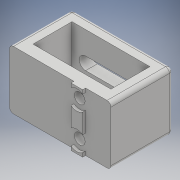
# Autodesk Inventor part: Estrutura - Suporte Mesa
Saved by Autodesk Inventor 2017 (Build 210142000, 142)
## iProperties
Created: 2020-08-23
Part Number: Estrutura - Suporte Mesa
Material: Generic
Document SubType Name: Modeling
Designer: ale
Density: 1 g/cm^3
Appearance: Default
Author: ale
Autodesk Inventor part; units mm, degrees
note: some values were not read from the file. Chosen so that the rebuilt part matches the saved one: direction of "Hole1".
ref_plane "YZ Plane" through (0, 0, 0) normal (1, 0, 0) x (0, 1, 0)
ref_plane "XZ Plane" through (0, 0, 0) normal (0, 1, 0) x (-1, 0, 0)
ref_plane "XY Plane" through (0, 0, 0) normal (0, 0, 1) x (1, 0, 0)
sketch "Sketch1" plane through (0, 0, 0) normal (0, 0, 1) x (1, 0, 0)
  line L0 (-12.2491, 0) -> (12.2491, 0)
  line L1 (0, 10.917) -> (0, -10.917)
  line L2 (-30, -10) -> (-30, -16)
  line L3 (-30, -16) -> (16, -16)
  line L4 (-30, -10) -> (10, -10)
  line L5 (10, -10) -> (10, 10)
  line L6 (10, 10) -> (-30, 10)
  line L7 (-30, 10) -> (-30, 16)
  line L8 (-30, 16) -> (16, 16)
  line L9 (16, 16) -> (16, -16)
  point P0 (0, 0)
  point P1 (0, 0)
  dimension "d0" = 10
  dimension "d1" = 10
  dimension "d2" = 10
  dimension "d3" = 30
  dimension "d4" = 6
  dimension "d5" = 6
  dimension "d6" = 40
  dimension "d7" = 6
  constraints: 20 end point, 6 perpendicular, 2 horizontal, 2 midpoint, 2 vertical, 1 coincident
  measures "d0" distance between parallel lines of L6 L0
  measures "d1" distance between parallel lines of L4 L0
  measures "d2" distance between parallel lines of L5 L1
  measures "d3" distance between parallel lines of L2 L1
  measures "d4" distance between parallel lines of L3 L4
  measures "d5" distance between parallel lines of L9 L5
  measures "d6" distance between parallel lines of L7 L5
  measures "d7" distance between parallel lines of L6 L8
extrude "Extrusion1" add sketch "Sketch1" along normal blind 30 contours L5 L6 L7 L8 L9 L3 L2 L4
sketch "Sketch2" plane through (-30, -16, 0) normal (0, -1, 0) x (1, 0, 0)
  line L0 (40, 30) -> (0, 30) projected
  line L1 (27, 30) -> (27, 0)
  line L2 (0, 0) -> (0, 30) projected
  line L3 (33, 30) -> (33, 0)
  line L4 (40, 0) -> (0, 0) projected
  line L5 (27, 30) -> (33, 30)
  line L6 (33, 0) -> (27, 0)
  line L7 (46, 0) -> (46, 30) projected
  line L8 (40, 0) -> (40, 30) projected
  point P0 (30, 0)
  dimension "d37" = 13
  dimension "d38" = 7
  constraints: 8 end point, 3 point on line, 2 collinear, 1 perpendicular, 1 vertical
  measures "d37" distance between parallel lines of L8 L1
  measures "d38" distance between parallel lines of L8 L3
extrude "Extrusion2" add sketch "Sketch2" along normal blind 1.5 contours L3 L4 L1 L0
sketch "Sketch3" plane through (-30, -17.5, 0) normal (0, -1, 0) x (1, 0, 0)
  line L0 (27, 0) -> (33, 0) projected
  line L1 (27, 30) -> (27, 0) projected
  line L2 (27, 15) -> (13, 15)
  line L3 (33, 0) -> (33, 30) projected
  point P0 (30, 0)
  point P1 (30, 6)
  point P2 (30, 24)
  dimension "d14" = 6
  dimension "d36" = 3
  constraints: 2 end point, 1 horizontal, 1 midpoint, 1 symmetric about line
  measures "d14" distance from line of L0 point (30, 6)
  measures "d36" distance from line of L3 point (30, 6)
hole "Hole1" at (0, -17.5, 6) at (0, -17.5, 24) direction (0, 1, 0) diameter 5.5 end up to surface counterbore diameter 10 counterbore depth 1.5
sketch "Sketch4" plane through (-30, 16, 0) normal (0, 1, 0) x (1, 0, 0)
  arc A0 (7, -11.75) -> (7, -18.25) centre (7, -15) ccw
  line L0 (0, 0) -> (0, -30) projected
  line L1 (46, 0) -> (0, 0) projected
  arc A1 (34, -18.25) -> (34, -11.75) centre (34, -15) ccw
  line L2 (46, -30) -> (0, -30) projected
  line L3 (34, -11.75) -> (7, -11.75)
  line L4 (34, -18.25) -> (7, -18.25)
  point P0 (30, 0)
  dimension "d22" = 6.5
  dimension "d23" = 7
  dimension "d24" = 15
  dimension "d25" = 6.5
  dimension "d26" = 34
  dimension "d27" = 15
  constraints: 4 end point, 4 point on circle, 4 tangent, 2 centre point
  measures "d22" diameter of A0
  measures "d23" distance from line of L0 A0.centre
  measures "d24" distance from line of L1 A0.centre
  measures "d25" diameter of A1
  measures "d26" distance from line of L0 A1.centre
  measures "d27" distance from line of L2 A1.centre
extrude "Extrusion3" cut sketch "Sketch4" against normal up to surface (6 mm away)
sketch "Sketch5" plane through (-30, -16, 0) normal (-1, 0, 0) x (0, 0, 1)
  line L0 (0, 0) -> (0, 32) projected
  line L1 (30, 6) -> (30, 0) projected
  line L2 (0, 32) -> (30, 32)
  line L3 (30, 32) -> (30, 0)
  line L4 (30, 0) -> (0, 0)
  line L5 (0, 0) -> (0, 32)
  point P0 (0, 16)
  constraints: 8 end point, 2 parallel, 1 horizontal, 1 perpendicular
extrude "Extrusion4" add sketch "Sketch5" along normal blind 6
fillet "Fillet3" radius 2 8 edges at (16, 0, 30) (-10, 16, 30) (-36, 16, 15) (-36, 0, 30) (-36, 0, 0) (-10, 16, 0) (16, 16, 15) (16, 0, 0)
body "Solid1"
